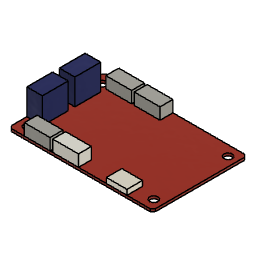
总线舵机信号转换版 v2 (Autodesk Fusion 360 design; units mm, degrees)
Autodesk Fusion 360 part; units mm, degrees
sketch "草图1" plane through (0, 0, 0) normal (0, 0, 1) x (1, 0, 0)
  line L0 (1, 0) -> (54.8, 0)
  line L1 (55.8, 1) -> (55.8, 35.6)
  line L2 (54.8, 36.6) -> (1, 36.6)
  line L3 (0, 35.6) -> (0, 1)
  line L4 (-8.6099, 18.3) -> (78, 18.3)
  line L5 (27.9, 45) -> (27.9, -14)
  circle A0 centre (3.5, 32.7) radius 1.6
  circle A1 centre (52.3, 32.7) radius 1.6
  circle A2 centre (3.5, 3.9) radius 1.6
  circle A3 centre (52.3, 3.9) radius 1.6
  line L6 (55.8, 35.6) -> (54.8, 36.6)
  line L7 (54.8, 0) -> (55.8, 1)
  line L8 (1, 36.6) -> (0, 35.6)
  line L9 (1, 0) -> (0, 1)
  point P0 (55.8, 0)
  point P1 (55.8, 36.6)
  point P2 (0, 36.6)
  dimension "d1" = 55.8
  dimension "d2" = 36.6
  dimension "d3" = 3.2
  dimension "d4" = 48.8
  dimension "d5" = 28.8
  dimension "d6" = 1
  dimension "d7" = 1
  dimension "d8" = 1
  dimension "d9" = 1
  dimension "d10" = 1
  dimension "d11" = 1
  dimension "d12" = 1
  dimension "d13" = 1
  constraint horizontal L0
  constraint vertical L1
  constraint horizontal L2
  constraint vertical L3
  constraint perpendicular L3 L4
  constraint perpendicular L0 L5
  constraint symmetric L5 A0 A1
  constraint symmetric L4 A0 A2
  constraint symmetric L4 A1 A3
  constraint coincident P1 L1
  constraint coincident P1 L2
  constraint coincident P0 L0
  constraint coincident P0 L1
  constraint coincident P2 L2
  constraint coincident P2 L3
  constraint coincident origin L0
  constraint coincident origin L3
  measures "d1" distance of P1 P2
  measures "d2" distance of origin P2
  measures "d3" diameter of A0
  measures "d4" distance of A0.centre A1.centre
  measures "d5" distance of A0.centre A2.centre
  measures "d6" distance of P1 L1.end
  measures "d7" distance of P1 L2.start
  measures "d8" distance of P0 L0.end
  measures "d9" distance of P0 L1.start
  measures "d10" distance of P2 L2.end
  measures "d11" distance of P2 L3.start
  measures "d12" distance of origin L0.start
  measures "d13" distance of origin L3.end
extrude "拉伸1" add sketch "草图1" along normal blind 1 makes body 1
sketch "草图2" plane through (0, 0, 1) normal (0, 0, 1) x (-1, 0, 0)
  circle A0 centre (-3.5, -3.9) radius 1.6
  circle A1 centre (-52.3, -32.7) radius 1.6
  circle A2 centre (-3.5, -32.7) radius 1.6
  circle A3 centre (-52.3, -3.9) radius 1.6
  line L0 (-54.8, 0) -> (-55.8, -1)
  line L1 (-55.8, -1) -> (-55.8, -35.6)
  line L2 (-55.8, -35.6) -> (-54.8, -36.6)
  line L3 (-54.8, -36.6) -> (-1, -36.6)
  line L4 (-1, -36.6) -> (0, -35.6)
  line L5 (0, -35.6) -> (0, -1)
  line L6 (0, -1) -> (-1, 0)
  line L7 (-1, 0) -> (-54.8, 0)
  line L8 (0, -29.6) -> (-6, -29.6)
  line L9 (-6, -29.6) -> (-6, -19.6)
  line L10 (-6, -19.6) -> (0, -19.6)
  line L11 (0, -19.6) -> (0, -29.6)
  line L12 (0, -17) -> (-6, -17)
  line L13 (-6, -17) -> (-6, -7)
  line L14 (-6, -7) -> (0, -7)
  line L15 (0, -7) -> (0, -17)
  dimension "d16" = 6
  dimension "d17" = 6
  dimension "d18" = 10
  dimension "d19" = 10
  dimension "d20" = 7
  dimension "d21" = 7
  constraint horizontal L8
  constraint vertical L9
  constraint horizontal L10
  constraint vertical L11
  constraint coincident L5 L8.start
  constraint horizontal L12
  constraint vertical L13
  constraint horizontal L14
  constraint vertical L15
  measures "d16" distance of L8.start L8.end
  measures "d17" distance of L12.start L12.end
  measures "d18" distance of L8.end L9.end
  measures "d19" distance of L12.end L13.end
  measures "d20" distance of L3 L8
  measures "d21" distance of L7 L14
extrude "拉伸2" add sketch "草图2" along normal blind 10 separate body contours L5 L12 L13 L14 L15 | L5 L8 L9 L10 L11 makes body 2 at (0, 13.6667, 4.3333) makes body 3 at (0, 26.2667, 4.3333)
sketch "草图3" plane through (0, 0, 1) normal (0, 0, 1) x (-1, 0, 0)
  circle A0 centre (-3.5, -3.9) radius 1.6
  circle A1 centre (-52.3, -32.7) radius 1.6
  circle A2 centre (-3.5, -32.7) radius 1.6
  circle A3 centre (-52.3, -3.9) radius 1.6
  line L0 (-54.8, 0) -> (-55.8, -1)
  line L1 (-55.8, -1) -> (-55.8, -35.6)
  line L2 (-55.8, -35.6) -> (-54.8, -36.6)
  line L3 (-54.8, -36.6) -> (-1, -36.6)
  line L4 (-1, -36.6) -> (0, -35.6)
  line L5 (0, -35.6) -> (0, -1)
  line L6 (0, -1) -> (-1, 0)
  line L7 (-1, 0) -> (-54.8, 0)
  line L8 (-6, -36.6) -> (-16, -36.6)
  line L9 (-16, -36.6) -> (-16, -31.6)
  line L10 (-16, -31.6) -> (-6, -31.6)
  line L11 (-6, -31.6) -> (-6, -36.6)
  line L12 (-17, -36.6) -> (-27, -36.6)
  line L13 (-27, -36.6) -> (-27, -31.6)
  line L14 (-27, -31.6) -> (-17, -31.6)
  line L15 (-17, -31.6) -> (-17, -36.6)
  line L16 (-6, 0) -> (-16, 0)
  line L17 (-16, 0) -> (-16, -5)
  line L18 (-16, -5) -> (-6, -5)
  line L19 (-6, -5) -> (-6, 0)
  line L20 (-17, 0) -> (-27, 0)
  line L21 (-27, 0) -> (-27, -5)
  line L22 (-27, -5) -> (-17, -5)
  line L23 (-17, -5) -> (-17, 0)
  dimension "d24" = 5
  dimension "d25" = 5
  dimension "d26" = 5
  dimension "d27" = 5
  dimension "d28" = 10
  dimension "d29" = 10
  dimension "d30" = 10
  dimension "d31" = 10
  dimension "d32" = 6
  dimension "d33" = 6
  dimension "d34" = 1
  dimension "d35" = 1
  constraint horizontal L8
  constraint vertical L9
  constraint horizontal L10
  constraint vertical L11
  constraint coincident L3 L8.start
  constraint horizontal L12
  constraint vertical L13
  constraint horizontal L14
  constraint vertical L15
  constraint coincident L3 L12.start
  constraint horizontal L16
  constraint vertical L17
  constraint horizontal L18
  constraint vertical L19
  constraint coincident L7 L16.start
  constraint horizontal L20
  constraint vertical L21
  constraint horizontal L22
  constraint vertical L23
  constraint coincident L7 L20.start
  measures "d24" distance of L8.start L10.end
  measures "d25" distance of L12.end L13.end
  measures "d26" distance of L16.start L18.end
  measures "d27" distance of L20.end L21.end
  measures "d28" distance of L8.start L8.end
  measures "d29" distance of L12.start L12.end
  measures "d30" distance of L16.start L16.end
  measures "d31" distance of L20.start L20.end
  measures "d32" distance of L5 L11
  measures "d33" distance of L5 L19
  measures "d34" distance of L9 L15
  measures "d35" distance of L17 L23
extrude "拉伸3" add sketch "草图3" along normal blind 4.5 separate body contours L7 L20 L21 L22 L23 | L7 L16 L17 L18 L19 | L3 L12 L13 L14 L15 | L3 L8 L9 L10 L11 makes body 4 at (23.6667, 33.2667, 1) makes body 5 at (9.3333, 3.3333, 1) makes body 6 at (12.6667, 33.2667, 1) makes body 7 at (23.6667, 3.3333, 1)
sketch "草图4" plane through (0, 0, 1) normal (0, 0, 1) x (-1, 0, 0)
  circle A0 centre (-3.5, -3.9) radius 1.6
  circle A1 centre (-52.3, -32.7) radius 1.6
  circle A2 centre (-3.5, -32.7) radius 1.6
  circle A3 centre (-52.3, -3.9) radius 1.6
  line L0 (-54.8, 0) -> (-55.8, -1)
  line L1 (-55.8, -1) -> (-55.8, -35.6)
  line L2 (-55.8, -35.6) -> (-54.8, -36.6)
  line L3 (-54.8, -36.6) -> (-1, -36.6)
  line L4 (-1, -36.6) -> (0, -35.6)
  line L5 (0, -35.6) -> (0, -1)
  line L6 (0, -1) -> (-1, 0)
  line L7 (-1, 0) -> (-54.8, 0)
  line L8 (-37.8, -6) -> (-45.8, -6)
  line L9 (-45.8, -6) -> (-45.8, 0)
  line L10 (-45.8, 0) -> (-37.8, 0)
  line L11 (-37.8, 0) -> (-37.8, -6)
  dimension "d38" = 8
  dimension "d39" = 6
  dimension "d40" = 10
  constraint horizontal L8
  constraint vertical L9
  constraint horizontal L10
  constraint vertical L11
  constraint coincident L7 L9.end
  measures "d38" distance of L8.start L8.end
  measures "d39" distance of L8.end L9.end
  measures "d40" distance of L1 L9
extrude "拉伸4" add sketch "草图4" along normal blind 2 separate body contours L7 L8 L9 L10 L11 makes body 8
copy_body "实体->零部件1" bodies 1 removing the originals makes body 9 in component "Component'"
copy_body "实体->零部件2" bodies 2 removing the originals makes body 10 in component "Component''"
copy_body "实体->零部件3" bodies 3 removing the originals makes body 11 in component "Component'''"
copy_body "实体->零部件4" bodies 4 removing the originals makes body 12 in component "Component''''"
copy_body "实体->零部件5" bodies 5 removing the originals makes body 13 in component "Component'''''"
copy_body "实体->零部件6" bodies 6 removing the originals makes body 14 in component "Component''''''"
copy_body "实体->零部件7" bodies 7 removing the originals makes body 15 in component "Component'''''''"
copy_body "实体->零部件8" bodies 8 removing the originals makes body 16 in component "Component''''''''"
component "Component'" placed x (1, 0, 0) y (0, 1, 0) z (0, 0, 1) at (0, 0, 0)
component "Component''" placed x (1, 0, 0) y (0, 1, 0) z (0, 0, 1) at (0, 0, 0)
component "Component'''" placed x (1, 0, 0) y (0, 1, 0) z (0, 0, 1) at (0, 0, 0)
component "Component''''" placed x (1, 0, 0) y (0, 1, 0) z (0, 0, 1) at (0, 0, 0)
component "Component'''''" placed x (1, 0, 0) y (0, 1, 0) z (0, 0, 1) at (0, 0, 0)
component "Component''''''" placed x (1, 0, 0) y (0, 1, 0) z (0, 0, 1) at (0, 0, 0)
component "Component'''''''" placed x (1, 0, 0) y (0, 1, 0) z (0, 0, 1) at (0, 0, 0)
component "Component''''''''" placed x (1, 0, 0) y (0, 1, 0) z (0, 0, 1) at (0, 0, 0)
equation "d7 = d6"
equation "d9 = d8"
equation "d11 = d10"
equation "d13 = d12"
